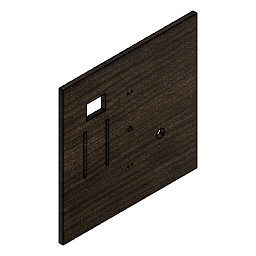
plate (Autodesk Fusion 360 design; units mm, degrees)
part number: 2026-06-01-11-50-28-145
Autodesk Fusion 360 part; units mm, degrees
sketch "Plate" plane through (0, 0, 0) normal (1, 0, 0) x (0, 1, 0)
  line L0 (95, 95) -> (-95, 95)
  line L1 (-95, 95) -> (-95, -95)
  line L2 (-95, -95) -> (95, -95)
  line L3 (95, -95) -> (95, 95)
  line L4 (95, 95) -> (-95, -95) construction
  line L5 (-95, 95) -> (95, -95) construction
  line L6 (90, -90) -> (90, 90)
  line L7 (90, 90) -> (-90, 90)
  line L8 (-90, 90) -> (-90, -90)
  line L9 (-90, -90) -> (90, -90)
  line L10 (85, -85) -> (85, 85)
  line L11 (85, 85) -> (-85, 85)
  line L12 (-85, 85) -> (-85, -85)
  line L13 (-85, -85) -> (85, -85)
  circle A0 centre (0, 0) radius 2.5
  line L14 (-55, 55) -> (-31, 55)
  line L15 (-31, 55) -> (-31, 36)
  line L16 (-31, 36) -> (-55, 36)
  line L17 (-55, 36) -> (-55, 55)
  line L18 (-57.0845, 85) -> (-57.0845, -85) construction
  line L19 (-28.9155, 85) -> (-28.9155, -85) construction
  line L20 (-55.5845, 25) -> (-58.5845, 25)
  line L21 (-58.5845, 25) -> (-58.5845, -25)
  line L22 (-58.5845, -25) -> (-55.5845, -25)
  line L23 (-55.5845, -25) -> (-55.5845, 25)
  line L24 (-85, 0) -> (85, 0) construction
  line L25 (-30.3955, 25) -> (-30.3955, -25)
  line L26 (-27.3955, -25) -> (-27.3955, 25)
  line L27 (-30.3955, -25) -> (-27.3955, -25)
  line L28 (-27.3955, 25) -> (-30.3955, 25)
  line L29 (0, 85) -> (0, -85) construction
  circle A1 centre (38.833, -24.365) radius 5
  circle A2 centre (-2.3875, 40) radius 1
  circle A3 centre (2.3875, 40) radius 1
  circle A4 centre (-2.3875, -40) radius 1
  circle A5 centre (2.3875, -40) radius 1
  line L30 (-43, 0) -> (-43, -9.5) construction
  line L31 (-43, 0) -> (-43, 9.5) construction
  dimension "d1" = 190
  dimension "d2" = 190
  dimension "d3" = -5
  dimension "d4" = -5
  dimension "d5" = 5
  dimension "d6" = 24
  dimension "d7" = 19
  dimension "d8" = 30
  dimension "d9" = 30
  dimension "d10" = 28.169
  dimension "d11" = 2.0845
  dimension "d12" = 50
  dimension "d13" = 3
  dimension "d14" = 1.5
  dimension "d15" = 25
  dimension "d16" = 50
  dimension "d17" = 3
  dimension "d18" = 25.189
  dimension "d19" = 25
  dimension "d29" = 10
  dimension "d30" = 24.365
  dimension "d31" = 38.833
  dimension "d35" = 2
  dimension "d36" = 2
  dimension "d37" = 4.775
  dimension "d38" = 40
  dimension "d39" = 2.3875
  dimension "d40" = 40
  dimension "d41" = 9.5
  dimension "d42" = 9.5
  constraint horizontal L0
  constraint perpendicular L0 L1
  constraint parallel L0 L2
  constraint parallel L1 L3
  constraint coincident L4 A0.centre
  constraint coincident L5 A0.centre
  constraint coincident A0.centre origin
  constraint horizontal L14
  constraint vertical L15
  constraint horizontal L16
  constraint vertical L17
  constraint coincident L11 L18.start
  constraint coincident L13 L18.end
  constraint perpendicular L13 L18
  constraint coincident L11 L19.start
  constraint coincident L13 L19.end
  constraint perpendicular L13 L19
  constraint horizontal L20
  constraint vertical L21
  constraint horizontal L22
  constraint vertical L23
  constraint midpoint L12 L24.start
  constraint midpoint L10 L24.end
  constraint horizontal L28
  constraint vertical L25
  constraint horizontal L27
  constraint vertical L26
  constraint midpoint L11 L29.start
  constraint midpoint L13 L29.end
  constraint symmetric L24 A2 A4
  constraint symmetric L24 A3 A5
  constraint coincident L24 L30.start
  constraint perpendicular L24 L30
  constraint perpendicular L24 L31
  measures "d1" distance of L1.end L2.end
  measures "d2" distance of L0.end L1.end
  measures "d5" diameter of A0
  measures "d6" distance of L14.start L14.end
  measures "d7" distance of L14.start L16.end
  measures "d8" distance of L12 L17
  measures "d9" distance of L11 L14
  measures "d10" distance of L18 L19
  measures "d11" distance of L15 L19
  measures "d12" distance of L20.end L21.end
  measures "d13" distance of L21 L23
  measures "d14" distance of L18 L23
  measures "d15" distance of L20 L24
  measures "d16" distance of L25.end L25.start
  measures "d17" distance of L25 L26
  measures "d18" distance of L23 L25
  measures "d19" distance of L24 L28
  measures "d29" diameter of A1
  measures "d30" distance of L24 A1.centre
  measures "d31" distance of L29 A1.centre
  measures "d35" diameter of A2
  measures "d36" diameter of A3
  measures "d37" horizontal distance of A2.centre A3.centre
  measures "d38" distance of L24 A2.centre
  measures "d39" distance of L29 A2.centre
  measures "d40" distance of L24 A3.centre
  measures "d41" distance of L30.start L30.end
  measures "d42" distance of L30.start L31.end
extrude "Extrude1" add sketch "Plate" along normal mid plane 5 contours L10 L11 L12 L13
equation "d2 = d1"
equation "d8 = ( 30 * d1 / 190 mm ) * 1 mm"
equation "d9 = ( 30 * d1 / 190 mm ) * 1 mm"
equation "d11 = ( ( 28.169 - 24 ) / 2 ) * 1 mm"
equation "d16 = d12"
equation "d17 = d13"
equation "d19 = d15"
equation "d39 = ( 4.775 / 2 ) * 1 mm"
